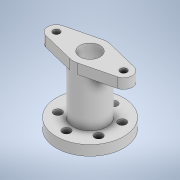
# Autodesk Inventor part: Exercise05
Saved by Autodesk Inventor 2021 (Build 250183000, 183)
## iProperties
Created: 2022-03-22
Part Number: Exercise05
Material: Generic
Document SubType Name: Modeling
Designer: User
Density: 1 g/cm^3
Appearance: Default
Author: User
Autodesk Inventor part; units mm, degrees
ref_plane "YZ Plane" through (0, 0, 0) normal (1, 0, 0) x (0, 1, 0)
ref_plane "XZ Plane" through (0, 0, 0) normal (0, 1, 0) x (-1, 0, 0)
ref_plane "XY Plane" through (0, 0, 0) normal (0, 0, 1) x (1, 0, 0)
sketch "Sketch1" plane through (0, 0, 0) normal (0, 1, 0) x (-1, 0, 0)
  circle A0 centre (0, 0) radius 50
  circle A1 centre (0, 0) radius 15
  circle A2 centre (0, 0) radius 35 construction
  circle A3 centre (0, -35) radius 6
  circle A4 centre (30.3109, -17.5) radius 6
  circle A5 centre (30.3109, 17.5) radius 6
  circle A6 centre (0, 35) radius 6
  circle A7 centre (-30.3109, 17.5) radius 6
  circle A8 centre (-30.3109, -17.5) radius 6
  dimension "d2" = 70
  dimension "d0" = 100
  dimension "d1" = 30
  dimension "d3" = 12
  dimension "d6" = 360
  constraints: 8 centre point, 3 coincident, 2 vertical alignment, 15 other
  measures "d0" diameter of A0
  measures "d1" diameter of A1
  measures "d3" diameter of A3
extrude "Extrusion1" add sketch "Sketch1" along normal blind 15
sketch "Sketch2" plane through (0, 15, 0) normal (0, 1, 0) x (1, 0, 0)
  circle A0 centre (0, 0) radius 25
  circle A1 centre (0, 0) radius 15 projected
  dimension "d10" = 50
  constraints: 1 centre point, 1 coincident
  measures "d10" diameter of A0
extrude "Extrusion2" add sketch "Sketch2" along normal blind 70
sketch "Sketch3" plane through (0, 85, 0) normal (0, 1, 0) x (1, 0, 0)
  circle A0 centre (-50, 0) radius 13
  circle A1 centre (-50, 0) radius 5
  circle A2 centre (50, 0) radius 13
  circle A3 centre (50, 0) radius 5
  circle A4 centre (0, 0) radius 50 construction
  circle A5 centre (0, 0) radius 25 projected
  circle A6 centre (0, 0) radius 15 projected
  line L0 (-6, 24.2693) -> (-53.12, 12.62)
  line L1 (-6, -24.2693) -> (-53.12, -12.62)
  line L2 (6, 24.2693) -> (53.12, 12.62)
  line L3 (6, -24.2693) -> (53.12, -12.62)
  dimension "d13" = 26
  dimension "d14" = 10
  dimension "d15" = 26
  dimension "d16" = 10
  dimension "d17" = 100
  constraints: 8 end point, 8 point on circle, 8 tangent, 4 centre point, 3 horizontal alignment, 2 coincident, 1 other
  measures "d13" diameter of A0
  measures "d14" diameter of A1
  measures "d15" diameter of A2
  measures "d16" diameter of A3
  measures "d17" distance of A2.centre A0.centre
extrude "Extrusion3" add sketch "Sketch3" along normal blind 15
body "Solid1"
